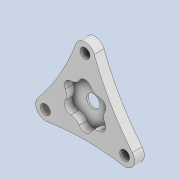
# Autodesk Inventor part: m0.5z80接続部品
Saved by Autodesk Inventor 2020.4 (Build 244396000, 396)
## iProperties
Created: 2021-04-23
Part Number: m0.5z80接続部品
Material: アルミニウム 2014-T4
Document SubType Name: Modeling
Designer: happy
Density: 2.8 g/cm^3
Appearance: サテン
Author: happy
Autodesk Inventor part; units mm, degrees
ref_plane "YZ Plane" through (0, 0, 0) normal (1, 0, 0) x (0, 1, 0)
ref_plane "XZ Plane" through (0, 0, 0) normal (0, 1, 0) x (-1, 0, 0)
ref_plane "XY Plane" through (0, 0, 0) normal (0, 0, 1) x (1, 0, 0)
sketch "スケッチ1" plane through (0, 0, 0) normal (0, 0, 1) x (1, 0, 0)
  circle A0 centre (0, 0) radius 18.25
  circle A1 centre (0, 0) radius 17
  line L0 (0, 14) -> (12.1244, -7) construction
  line L1 (12.1244, -7) -> (-12.1244, -7) construction
  line L2 (-12.1244, -7) -> (0, 14) construction
  circle A2 centre (0, 14) radius 1.5
  circle A3 centre (-12.1244, -7) radius 1.5
  circle A4 centre (12.1244, -7) radius 1.5
  circle A5 centre (0, 14) radius 3
  circle A6 centre (-12.1244, -7) radius 3
  circle A7 centre (12.1244, -7) radius 3
  circle A8 centre (0, 0) radius 8 construction
  circle A9 centre (0, 0) radius 7 construction
  line L3 (0, 7) -> (6.0622, 3.5) construction
  line L4 (6.0622, 3.5) -> (6.0622, -3.5) construction
  line L5 (6.0622, -3.5) -> (0, -7) construction
  line L6 (0, -7) -> (-6.0622, -3.5) construction
  line L7 (-6.0622, -3.5) -> (-6.0622, 3.5) construction
  line L8 (-6.0622, 3.5) -> (0, 7) construction
  arc A10 (1.7321, 6) -> (-1.7321, 6) centre (0, 5) ccw
  arc A11 (-4.3301, 4.5) -> (-6.0622, 1.5) centre (-4.3301, 2.5) ccw
  arc A12 (-6.0622, -1.5) -> (-4.3301, -4.5) centre (-4.3301, -2.5) ccw
  arc A13 (-1.7321, -6) -> (1.7321, -6) centre (0, -5) ccw
  arc A14 (4.3301, -4.5) -> (6.0622, -1.5) centre (4.3301, -2.5) ccw
  arc A15 (6.0622, 1.5) -> (4.3301, 4.5) centre (4.3301, 2.5) ccw
  arc A16 (1.7321, 6) -> (4.3301, 4.5) centre (4.3301, 7.5) ccw
  arc A17 (-4.3301, 4.5) -> (-1.7321, 6) centre (-4.3301, 7.5) ccw
  arc A18 (-6.0622, -1.5) -> (-6.0622, 1.5) centre (-8.6603, 0) ccw
  arc A19 (-1.7321, -6) -> (-4.3301, -4.5) centre (-4.3301, -7.5) ccw
  arc A20 (4.3301, -4.5) -> (1.7321, -6) centre (4.3301, -7.5) ccw
  arc A21 (6.0622, 1.5) -> (6.0622, -1.5) centre (8.6603, 0) ccw
  circle A22 centre (0, 0) radius 5.6603 construction
  arc A23 (-14.4416, -5.0946) -> (-2.8087, 15.0541) centre (-69.282, 40) ccw
  arc A24 (11.6328, -9.9595) -> (-11.6328, -9.9595) centre (0, -80) ccw
  arc A25 (2.8087, 15.0541) -> (14.4416, -5.0946) centre (69.282, 40) ccw
  circle A26 centre (0, 0) radius 9 construction
  circle A27 centre (0, 0) radius 2.025
  point P0 (-15.3265, -15.7621)
  point P1 (-6.0622, -3.5)
  point P2 (0, -7)
  point P3 (6.0622, -3.5)
  point P4 (6.0622, 3.5)
  point P5 (-1.7321, -6)
  point P6 (-4.3301, -4.5)
  point P7 (-6.0622, -1.5)
  point P8 (-6.0622, 1.5)
  point P9 (-4.3301, 4.5)
  point P10 (6.0622, 1.5)
  point P11 (6.0622, -1.5)
  point P12 (4.3301, -4.5)
  point P13 (1.7321, -6)
  point P14 (-11.6328, -9.9595)
  point P15 (11.6328, -9.9595)
  point P16 (14.4416, -5.0946)
  point P17 (2.8087, 15.0541)
  dimension "d4" = 6
  dimension "d5" = 6
  dimension "d13" = 14
  dimension "d0" = 34
  dimension "d1" = 3
  dimension "d2" = 3
  dimension "d3" = 3
  dimension "d6" = 6
  dimension "d7" = 14
  dimension "d12" = 16
  dimension "d14" = 360
  dimension "d15" = 360
  dimension "d16" = 11.3205
  dimension "d17" = 3
  dimension "d18" = 2
  dimension "d21" = 360
  dimension "d23" = 18
  dimension "d28" = 4.05
  constraints: 36 point on circle, 25 centre point, 18 end point, 14 coincident, 3 tangent, 2 point on line, 1 horizontal, 1 vertical, 1 vertical alignment, 102 other
  measures "d0" diameter of A1
  measures "d1" diameter of A2
  measures "d2" diameter of A3
  measures "d3" diameter of A4
  measures "d6" diameter of A7
  measures "d7" distance of A0.centre L0.start
  measures "d12" diameter of A8
  measures "d16" diameter of A22
  measures "d17" radius of A16
  measures "d18" radius of A10
  measures "d23" diameter of A26
  measures "d28" diameter of A27
extrude "押し出し1" add sketch "スケッチ1" along normal blind 3 contours A5 | A7 | A6 | A25 A7 A24 A6 A23 A5
extrude "押し出し2" add sketch "スケッチ1" along normal blind 0.5 contours A16 A15 A21 A14 A20 A13 A19 A12 A18 A11 A17 A10
